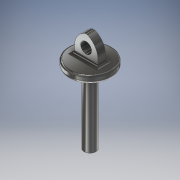
# Autodesk Inventor part: Part4
Saved by Autodesk Inventor 2019 (Build 230136000, 136)
## iProperties
Created: 2021-05-14
Part Number: Part4
Material: Generic
Document SubType Name: Modeling
Designer: HP
Density: 1 g/cm^3
Appearance: Default
Author: HP
Autodesk Inventor part; units mm, degrees
ref_plane "YZ Plane" through (0, 0, 0) normal (1, 0, 0) x (0, 1, 0)
ref_plane "XZ Plane" through (0, 0, 0) normal (0, 1, 0) x (-1, 0, 0)
ref_plane "XY Plane" through (0, 0, 0) normal (0, 0, 1) x (1, 0, 0)
sketch "Sketch1" plane through (0, 0, 0) normal (0, 0, 1) x (1, 0, 0)
  circle A0 centre (0, 0) radius 27.5
  dimension "d0" = 55
  constraints: 1 centre point, 1 coincident
  measures "d0" diameter of A0
extrude "Extrusion1" add sketch "Sketch1" along normal blind 10
sketch "Sketch2" plane through (0, 0, 10) normal (0, 0, 1) x (1, 0, 0)
  circle A0 centre (0, 0) radius 7.5
  dimension "d3" = 15
  constraints: 1 centre point, 1 coincident
  measures "d3" diameter of A0
extrude "Extrusion2" add sketch "Sketch2" along normal blind 90
fillet "Fillet1" radius 4 2 edges at (-7.5, 0, 10) (-27.5, 0, 10)
fillet "Fillet2" radius 2 1 edges at (-27.5, 0, 0)
sketch "Sketch3" plane through (0, 0, 0) normal (1, 0, 0) x (0, 1, 0)
  line L0 (25.5, 0) -> (-25.5, 0) projected
  line L1 (-15, 0) -> (-15, -10)
  arc A0 (-15, -10) -> (-2.0849, -29.1684) centre (7.1684, -8.9987) ccw
  line L2 (15, 0) -> (15, -10)
  arc A1 (2.0849, -29.1684) -> (15, -10) centre (-7.1684, -8.9987) ccw
  arc A2 (-2.0849, -29.1684) -> (2.0849, -29.1684) centre (0, -24.6238) ccw
  circle A3 centre (0, -14.191) radius 7
  line L3 (15, 0) -> (-15, 0)
  point P0 (0, 0)
  dimension "d9" = 15
  dimension "d10" = 10
  dimension "d11" = 22.191
  dimension "d12" = 30
  dimension "d13" = 5
  dimension "d15" = 14
  constraints: 6 end point, 6 point on circle, 4 centre point, 2 tangent, 1 collinear, 1 perpendicular, 1 point on line
  measures "d9" distance of point (0, 0) L1.start
  measures "d10" distance of L1.start L1.end
  measures "d11" radius of A0
  measures "d12" distance between parallel lines of L1 L2
  measures "d13" radius of A2
  measures "d15" diameter of A3
extrude "Extrusion3" add sketch "Sketch3" along normal mid plane 10
fillet "Fillet3" radius 4 4 edges at (-5, 0, 0) (0, 15, 0) (5, 0, 0) (0, -15, 0)
body "Solid1"
